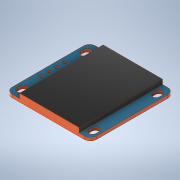
# Autodesk Inventor part: wishiot_oled
Saved by Autodesk Inventor 2020.2 (Build 242310000, 310)
## iProperties
Created: 2020-04-10
Part Number: wishiot_oled
Material: Phenolic Resin
Document SubType Name: Modeling
Designer: agmlego
Mass: 2.0467 g
Surface Area: 17.0385 cm^2
Volume: 1.48312 cm^3
Density: 1.38 g/cm^3
Appearance: Smooth - Light Orange
Author: agmlego
Autodesk Inventor part; units mm, degrees
ref_plane "YZ Plane" through (0, 0, 0) normal (1, 0, 0) x (0, 1, 0)
ref_plane "XZ Plane" through (0, 0, 0) normal (0, 1, 0) x (-1, 0, 0)
ref_plane "XY Plane" through (0, 0, 0) normal (0, 0, 1) x (1, 0, 0)
sketch "Sketch1" plane through (0, 0, 0) normal (0, 1, 0) x (-1, 0, 0)
  line L0 (2, 0) -> (25.3, 0)
  line L1 (27.3, -2) -> (27.3, -25)
  line L2 (25.3, -27) -> (2, -27)
  line L3 (0, -25) -> (0, -2)
  arc A0 (2, 0) -> (0, -2) centre (2, -2) ccw
  arc A1 (27.3, -2) -> (25.3, 0) centre (25.3, -2) ccw
  arc A2 (25.3, -27) -> (27.3, -25) centre (25.3, -25) ccw
  arc A3 (0, -25) -> (2, -27) centre (2, -25) ccw
  point P0 (0, 0)
  point P1 (27.3, 0)
  point P2 (0, -27)
  dimension "d0" = 27.3
  dimension "d1" = 27
  dimension "d2" = 2
  constraints: 8 end point, 8 point on circle, 8 tangent, 6 point on line, 4 centre point, 3 equal radius, 2 parallel, 1 horizontal, 1 perpendicular
  measures "d0" distance of point (0, 0) point (27.3, 0)
  measures "d1" distance of point (0, -27) point (0, 0)
  measures "d2" radius of A0
extrude "Extrusion1" add sketch "Sketch1" along normal blind 1
sketch "Sketch2" plane through (0, 1, 0) normal (0, 1, 0) x (1, 0, 0)
  arc A0 (-24.05, 24.075) -> (-26.3, 24.075) centre (-25.175, 24.075) ccw
  arc A1 (-26.3, 23.075) -> (-24.05, 23.075) centre (-25.175, 23.075) ccw
  line L0 (-26.3, 24.075) -> (-26.3, 23.075)
  line L1 (-24.05, 23.075) -> (-24.05, 24.075)
  line L2 (-27.3, 25) -> (-27.3, 2) projected
  line L3 (-2, 27) -> (-25.3, 27) projected
  arc A2 (-26.3, 2.575) -> (-24.05, 2.575) centre (-25.175, 2.575) ccw
  line L4 (-24.05, 2.575) -> (-24.05, 3.575)
  arc A3 (-24.05, 3.575) -> (-26.3, 3.575) centre (-25.175, 3.575) ccw
  line L5 (-26.3, 3.575) -> (-26.3, 2.575)
  arc A4 (-3.05, 23.075) -> (-0.8, 23.075) centre (-1.925, 23.075) ccw
  line L6 (-0.8, 23.075) -> (-0.8, 24.075)
  arc A5 (-0.8, 24.075) -> (-3.05, 24.075) centre (-1.925, 24.075) ccw
  line L7 (-3.05, 24.075) -> (-3.05, 23.075)
  arc A6 (-3.05, 2.575) -> (-0.8, 2.575) centre (-1.925, 2.575) ccw
  line L8 (-0.8, 2.575) -> (-0.8, 3.575)
  arc A7 (-0.8, 3.575) -> (-3.05, 3.575) centre (-1.925, 3.575) ccw
  line L9 (-3.05, 3.575) -> (-3.05, 2.575)
  point P0 (0, 0)
  dimension "d5" = 2.25
  dimension "d6" = 3.25
  dimension "d7" = 1
  dimension "d8" = 1.8
  dimension "d11" = 20.5
  dimension "d14" = 23.25
  constraints: 20 point on circle, 16 end point, 8 centre point, 4 point on line, 3 tangent, 2 vertical, 1 equal radius, 1 horizontal, 33 other
  measures "d5" distance between parallel lines of L1 L0
  measures "d7" distance between parallel lines of L2 L0
  measures "d8" distance edge to line of A0 L3
  measures "d11" distance of A1.centre A2.centre
  measures "d14" distance of A1.centre A4.centre
extrude "Extrusion2" cut sketch "Sketch2" against normal through all
sketch "Sketch3" plane through (0, 1, 0) normal (0, 1, 0) x (1, 0, 0)
  line L0 (-25.3, 0) -> (-2, 0) projected
  line L1 (-2, 27) -> (-25.3, 27) projected
  line L2 (-22.9, 0) -> (-3.7, 0)
  line L3 (-3.7, 0) -> (-3.7, 27)
  line L4 (-3.7, 27) -> (-22.9, 27)
  line L5 (-22.9, 27) -> (-22.9, 0)
  line L6 (-27.3, 25) -> (-27.3, 2) projected
  point P0 (0, 0)
  dimension "d19" = 19.2
  dimension "d20" = 4.4
  constraints: 8 end point, 2 parallel, 2 point on line, 1 horizontal, 1 perpendicular
  measures "d19" distance between parallel lines of L3 L5
  measures "d20" distance between parallel lines of L6 L5
extrude "Extrusion3" add sketch "Sketch3" along normal blind 1.5
sketch "Sketch4" plane through (0, 1, 0) normal (0, 1, 0) x (1, 0, 0)
  line L0 (-27.3, 25) -> (-27.3, 2) construction
  line L1 (-25.7, 12.23) -> (-27.3, 13.5) construction
  line L2 (-25.7, 14.77) -> (-27.3, 13.5) construction
  point P0 (0, 0)
  point P1 (-25.7, 9.69)
  point P2 (-25.7, 17.31)
  dimension "d25" = 2.54
  dimension "d30" = 1.6
  constraints: 4 end point, 1 equal length, 1 midpoint, 1 vertical, 3 other
  measures "d25" distance of point (-25.7, 9.69) L1.start
  measures "d30" distance from line of L0 point (-25.7, 9.69)
hole "Hole1" at (-25.7, 1, -9.69) at (-25.7, 1, -12.23) at (-25.7, 1, -14.77) at (-25.7, 1, -17.31) direction (0, -1, 0) diameter 1.016 end through all start extended yes
sketch "Sketch5" plane through (0, 0, 0) normal (0, -1, 0) x (1, 0, 0)
  circle A0 centre (-25.7, -9.69) radius 0.508 construction
sketch "Sketch6" plane through (0, 0, 0) normal (0, -1, 0) x (1, 0, 0)
  circle A0 centre (-25.7, -12.23) radius 0.508 construction
sketch "Sketch7" plane through (0, 0, 0) normal (0, -1, 0) x (1, 0, 0)
  circle A0 centre (-25.7, -14.77) radius 0.508 construction
sketch "Sketch8" plane through (0, 0, 0) normal (0, -1, 0) x (1, 0, 0)
  circle A0 centre (-25.7, -17.31) radius 0.508 construction
body "Solid1"
